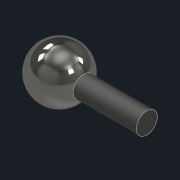
# Autodesk Inventor part: MCEN4000:T5
Saved by Autodesk Inventor 2021 (Build 250183000, 183)
## iProperties
Created: 2020-10-18
Part Number: MCEN4000:T5
Material: STEEL, AISI 1015
Document SubType Name: Modeling
Designer: Eugene Tang
Mass: 142.374 g
Surface Area: 41.7967 cm^2
Volume: 18.1368 cm^3
Density: 7.85 g/cm^3
Appearance: Black Metal
Description: TIE ROD OUTER BALL JOINT
Author: Eugene Tang
Autodesk Inventor part; units mm, degrees
ref_plane "YZ Plane" through (0, 0, 0) normal (1, 0, 0) x (0, 1, 0)
ref_plane "XZ Plane" through (0, 0, 0) normal (0, 1, 0) x (-1, 0, 0)
ref_plane "XY Plane" through (0, 0, 0) normal (0, 0, 1) x (1, 0, 0)
sketch "Sketch1" plane through (0, 0, 0) normal (0, 0, 1) x (1, 0, 0)
  circle A0 centre (-8.678, 43.8978) radius 15 construction
  line L0 (5.0697, 37.8978) -> (41.0697, 37.8978) construction
  line L1 (-28.678, 43.8978) -> (38.9288, 43.8978) construction
  line L2 (41.0697, 37.8978) -> (41.0697, 43.8978) construction
  line L3 (41.0697, 43.8978) -> (41.0697, 37.8978)
  line L4 (41.0697, 37.8978) -> (5.0697, 37.8978)
  line L5 (41.0697, 43.8978) -> (-23.678, 43.8978)
  arc A1 (-23.678, 43.8978) -> (5.0697, 37.8978) centre (-8.678, 43.8978) ccw
  point P0 (0, 0)
  point P1 (-23.678, 43.8978)
  constraints: 6 end point, 4 point on circle, 2 concentric, 2 perpendicular, 1 centre point, 1 point on line
revolve "Revolution1" add sketch "Sketch1" angle 360 about axis through (-28.678, 43.8978, 0) along (1, 0, 0)
body "Solid1"
